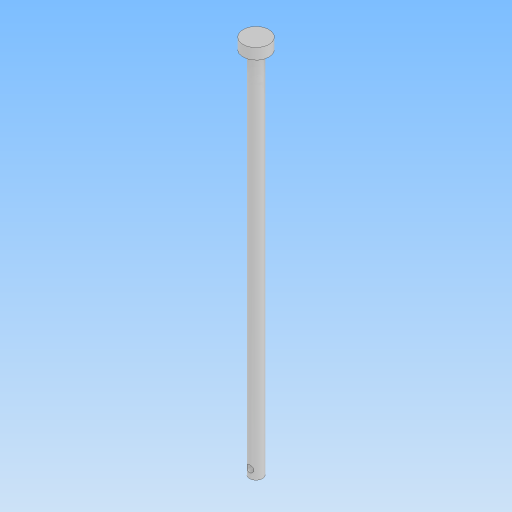
# Autodesk Inventor part: Bolzen fuer Ruder
Saved by Autodesk Inventor 2024.4 (Build 284460000, 460)
## iProperties
Created: 2026-01-22
Part Number: Bolzen fuer Ruder
Material: Generisch
Document SubType Name: Modeling
Designer: lucas
Mass: 5.32558 g
Surface Area: 36.5807 cm^2
Volume: 5.32558 cm^3
Density: 1 g/cm^3
Appearance: Vorgabe
Masse[kg]: 0,005 kg
Author: lucas
Autodesk Inventor part; units mm, degrees
ref_plane "YZ Plane" through (0, 0, 0) normal (1, 0, 0) x (0, 1, 0)
ref_plane "XZ Plane" through (0, 0, 0) normal (0, 1, 0) x (-1, 0, 0)
ref_plane "Arbeitsebene1" through (0, 0, 160) normal (0, 0, 1) x (1, 0, 0)
sketch "Skizze2" plane through (0, 0, 160) normal (0, 0, 1) x (1, 0, 0)
  circle A0 centre (0, 0) radius 6
  dimension "d3" = 12
  constraints: 1 centre point, 1 coincident
  measures "d3" diameter of A0
extrude "Extrusion2" add sketch "Skizze2" along normal blind 5
sketch "Skizze3" plane through (0, 0, 160) normal (0, 0, -1) x (-1, 0, 0)
  circle A0 centre (0, 0) radius 3
  dimension "d6" = 6
  constraints: 1 centre point, 1 coincident
  measures "d6" diameter of A0
extrude "Extrusion3" add sketch "Skizze3" along normal blind 170
sketch "Skizze4" plane through (0, 0, 0) normal (0, 1, 0) x (-1, 0, 0)
  line L0 (-3, -10) -> (3, -10) projected
  line L1 (0, -10) -> (0, 4)
  circle A0 centre (0, -6) radius 1.6
  point P0 (0, 0)
  dimension "d9" = 14
  dimension "d10" = 3.2
  constraints: 2 end point, 1 centre point, 1 midpoint, 1 point on line, 1 vertical
  measures "d9" distance of L1.start L1.end
  measures "d10" diameter of A0
extrude "Extrusion4" cut sketch "Skizze4" along normal mid plane 6
